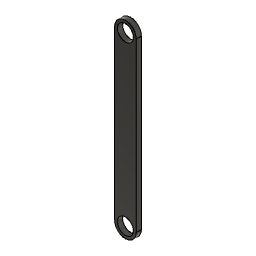
Coupler_B v3 (Autodesk Fusion 360 design; units mm, degrees)
Autodesk Fusion 360 part; units mm, degrees
sketch "Sketch1" plane through (0, 0, 0) normal (0, 1, 0) x (1, 0, 0)
  line L0 (-12.5, -96.75) -> (-12.5, 96.75)
  line L1 (12.5, 96.75) -> (12.5, -96.75)
  circle A0 centre (0, -96.75) radius 9.25
  arc A1 (-12.5, -96.75) -> (12.5, -96.75) centre (0, -96.75) ccw
  circle A2 centre (0, 96.75) radius 9.25
  arc A3 (12.5, 96.75) -> (-12.5, 96.75) centre (0, 96.75) ccw
  constraint parallel L0 L1
  constraint concentric A0 A1
extrude "Extrude1" add sketch "Sketch1" along normal blind 6
